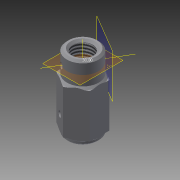
# Autodesk Inventor part: AnyaKicsi
Saved by Autodesk Inventor 2015 (Build 190159000, 159)
## iProperties
Created: 2014-08-26
Part Number: AnyaKicsi
Material: Generic
Document SubType Name: Modeling
Designer: laca
Density: 1 g/cm^3
Appearance: Default
Mass: 5.48937 g
Surface Area: 34.8539 cm^2
Volume: 5.48937 cm^3
Author: laca
Autodesk Inventor part; units mm, degrees
ref_plane "YZ Plane" through (0, 0, 0) normal (1, 0, 0) x (0, 1, 0)
ref_plane "XZ Plane" through (0, 0, 0) normal (0, 1, 0) x (-1, 0, 0)
ref_plane "XY Plane" through (0, 0, 0) normal (0, 0, 1) x (1, 0, 0)
sketch "Sketch1" plane through (0, 0, 0) normal (0, 1, 0) x (-1, 0, 0)
  line L0 (8.5475, 4.8243) -> (8.4517, -4.9902)
  line L1 (8.4517, -4.9902) -> (-0.0957, -9.8145)
  line L2 (-0.0957, -9.8145) -> (-8.5475, -4.8243)
  line L3 (-8.5475, -4.8243) -> (-8.4517, 4.9902)
  line L4 (-8.4517, 4.9902) -> (0.0957, 9.8145)
  line L5 (0.0957, 9.8145) -> (8.5475, 4.8243)
  circle A0 centre (0, 0) radius 5
  dimension "d0" = 17
  dimension "d1" = 10
  constraints: 12 end point, 2 coincident, 1 centre point, 13 other
  measures "d0" distance between parallel lines of L2 L5
  measures "d1" diameter of A0
extrude "Extrusion1" add sketch "Sketch1" along normal blind 37
sketch "Sketch2" plane through (0, 37, 0) normal (0, 1, 0) x (1, 0, 0)
  circle A0 centre (0, 0) radius 8
  circle A1 centre (0, 0) radius 13
  dimension "d4" = 16
  dimension "d5" = 5
  constraints: 2 centre point, 2 coincident
  measures "d4" diameter of A0
  measures "d5" radial gap between concentric circles of A1 A0
extrude "Extrusion2" cut sketch "Sketch2" against normal blind 12
sketch "Sketch3" plane through (0, 0, 0) normal (0, -1, 0) x (1, 0, 0)
  circle A0 centre (0, 0) radius 8
  circle A1 centre (0, 0) radius 13
  dimension "d9" = 16
  dimension "d10" = 5
  constraints: 2 centre point, 2 coincident
  measures "d9" diameter of A0
  measures "d10" radial gap between concentric circles of A1 A0
extrude "Extrusion3" cut sketch "Sketch3" against normal blind 3
chamfer "Chamfer1" distance 1 angle 45 6 edges at (-8, 3, 0) (-8, 0, 0) (5, 0, 0) (-8, 25, 0) (-8, 37, 0) (5, 37, 0)
ref_plane "Work Plane1" through (0, 31, 0) normal (0, 1, 0) x (1, 0, 0)
sketch "Sketch4" plane through (0, 31, 0) normal (0, 1, 0) x (1, 0, 0)
  line L0 (0, 0) -> (3.9142, 6.6294)
  line L1 (0.0957, 9.8145) -> (0, 0)
  point P0 (8.5475, 4.8243)
  dimension "d20" = 30
  constraints: 4 end point
  measures "d20" angle of L0 L1
ref_plane "Work Plane3" through (4.0674, 31, -6.8889) normal (0.5084234, 0, -0.8611072) x (0, 1, 0)
sketch "Sketch6" plane through (4.0674, 31, -6.8889) normal (0.5084234, 0, -0.8611072) x (0, 1, 0)
  circle A0 centre (0, 0) radius 1.5
  point P0 (-31, 0)
  dimension "d16" = 3
  constraints: 1 centre point
  measures "d16" diameter of A0
extrude "Extrusion4" cut sketch "Sketch6" against normal through all
sketch "Sketch9" plane through (0.0957, 3, -9.8145) normal (0.5084234, 0, -0.8611072) x (-0.8611072, 0, -0.5084234)
  circle A0 centre (-4.9075, 7) radius 1.5
  line L0 (-9.815, 0) -> (-9.815, 22) projected
  line L1 (0, 0) -> (0, 22) projected
  point P0 (-4.9075, -3)
  dimension "d31" = 3
  dimension "d32" = 9.8149
  dimension "d33" = 4.9075
  dimension "d34" = 10
  constraints: 1 centre point
  measures "d31" diameter of A0
  measures "d32" distance between parallel lines of L0 L1
  measures "d33" distance from line of L1 A0.centre
  measures "d34" distance of point (-4.907, -3) A0.centre
extrude "Extrusion5" cut sketch "Sketch9" against normal through all
thread "Thread2" size "M10x1.5" class "6H" standard "ANSI Metric M Profile" length 20
equation "\"d33\" = 0.5 * d32"
body "Solid1"
